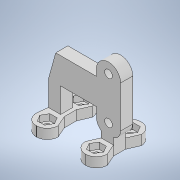
# Autodesk Inventor part: Крепление двигателя
Saved by Autodesk Inventor 2020 (Build 240168000, 168)
## iProperties
Created: 2021-05-24
Part Number: Крепление двигателя
Material: Типовые
Document SubType Name: Modeling
Designer: Антон
Density: 1 g/cm^3
Appearance: По умолчанию
Author: Антон
Autodesk Inventor part; units mm, degrees
ref_plane "YZ Plane" through (0, 0, 0) normal (1, 0, 0) x (0, 1, 0)
ref_plane "XZ Plane" through (0, 0, 0) normal (0, 1, 0) x (-1, 0, 0)
sketch "Эскиз1" plane through (0, 0, 0) normal (0, 0, 1) x (1, 0, 0)
  line L0 (0, 0) -> (26.75, 0)
  line L1 (26.75, 0) -> (26.75, 26)
  line L2 (26.75, 26) -> (0, 26)
  line L3 (0, 26) -> (0, 0)
  line L4 (0, 0) -> (16.75, 0)
  line L5 (16.75, 0) -> (16.75, 7.6)
  line L6 (16.75, 7.6) -> (0, 7.6)
  line L7 (0, 7.6) -> (0, 0)
  line L8 (0, 26) -> (16.75, 26)
  line L9 (16.75, 26) -> (16.75, 18.4)
  line L10 (16.75, 18.4) -> (0, 18.4)
  line L11 (0, 18.4) -> (0, 26)
  point P0 (0, 7.6)
  dimension "d0" = 26.75
  dimension "d1" = 26
  dimension "d14" = 16.75
  dimension "d15" = 7.6
  constraints: 24 end point, 6 parallel, 3 horizontal, 3 perpendicular, 2 equal length
  measures "d0" distance of L2.end L1.end
  measures "d1" distance of L1.end L0.end
  measures "d14" distance of L6.end L5.end
  measures "d15" distance of L5.end L4.end
extrude "Выдавливание1" add sketch "Эскиз1" along normal blind 5 contours L5 L6 L3 L10 L9 L2 L1 L0
sketch "Эскиз2" plane through (0, 0, 5) normal (0, 0, 1) x (1, 0, 0)
  line L0 (26.75, 0) -> (26.75, 26) projected
  line L1 (26.75, 13) -> (21.75, 13)
  line L2 (21.75, 13) -> (21.75, 21.75)
  line L3 (21.75, 13) -> (21.75, 4.25)
  point P0 (0, 0)
  dimension "d4" = 5
  dimension "d6" = 17.5
  constraints: 6 end point, 1 collinear, 1 horizontal, 1 midpoint, 1 perpendicular, 1 vertical
  measures "d4" distance of L1.start L1.end
  measures "d6" distance of L3.end L2.end
hole "Отверстие1" at (21.75, 21.75, 5) at (21.75, 4.25, 5) direction (0, 0, -1) diameter 3.2 end through all
sketch "Эскиз4" plane through (0, 0, 0) normal (0, 0, -1) x (-1, 0, 0)
  line L0 (-23.75, 0) -> (-18.75, 0)
  line L1 (-18.75, 0) -> (-18.75, -6.62)
  line L2 (-18.75, -6.62) -> (-23.75, -6.62)
  line L3 (-23.75, -6.62) -> (-23.75, 0)
  line L4 (3, 7.6) -> (-2, 7.6)
  line L5 (-2, 7.6) -> (-2, -6.62)
  line L6 (-2, -6.62) -> (3, -6.62)
  line L7 (3, -6.62) -> (3, 7.6)
  line L8 (-16.75, 0) -> (-26.75, 0) projected
  line L9 (-26.75, 0) -> (-26.75, 26) projected
  line L10 (0, 7.6) -> (-16.75, 7.6) projected
  line L11 (0, 18.4) -> (0, 7.6) projected
  point P0 (0, 0)
  dimension "d20" = 5
  dimension "d21" = 6.62
  dimension "d22" = 5
  dimension "d82" = 3
  dimension "d83" = 3
  constraints: 16 end point, 4 parallel, 3 collinear, 2 horizontal, 2 perpendicular
  measures "d20" distance of L1.end L2.end
  measures "d21" distance of L0.end L1.end
  measures "d22" distance of L6.end L5.end
  measures "d82" distance between parallel lines of L3 L9
  measures "d83" distance between parallel lines of L11 L7
extrude "Выдавливание3" add sketch "Эскиз4" against normal up to surface (5 mm away)
sketch "Эскиз5" plane through (18.75, -6.62, 0) normal (0, -1, 0) x (1, 0, 0)
  line L0 (7, 0) -> (-2, 0)
  line L1 (-2, 0) -> (-2, -9)
  line L2 (-2, -9) -> (7, -9)
  line L3 (7, -9) -> (7, 0)
  line L4 (5, 0) -> (0, 0) projected
  line L5 (-13.25, 0) -> (-22.25, 0)
  line L6 (-22.25, 0) -> (-22.25, -9)
  line L7 (-22.25, -9) -> (-13.25, -9)
  line L8 (-13.25, -9) -> (-13.25, 0)
  line L9 (-16.75, 0) -> (-18.75, 0) projected
  line L10 (-2, -4.5) -> (7, -4.5)
  line L11 (-13.25, -4.5) -> (-22.25, -4.5)
  circle A0 centre (-17.75, -4.5) radius 1.6
  circle A1 centre (2.5, -4.5) radius 1.6
  point P0 (2.5, 0)
  point P1 (-17.75, 0)
  dimension "d25" = 9
  dimension "d26" = 9
  dimension "d27" = 9
  dimension "d28" = 9
  dimension "d64" = 3.2
  dimension "d65" = 3.2
  constraints: 20 end point, 10 midpoint, 4 parallel, 2 centre point, 2 horizontal, 2 perpendicular
  measures "d25" distance of L2.end L1.end
  measures "d26" distance of L1.end L0.end
  measures "d27" distance of L7.end L6.end
  measures "d28" distance of L6.end L5.end
  measures "d64" diameter of A0
  measures "d65" diameter of A1
extrude "Выдавливание4" add sketch "Эскиз5" against normal blind 4 contours L3 L10 A1 L1 L0 | L3 L2 L1 L10 A1 | L8 L11 A0 L6 L5 | L8 L7 L6 L11 A0
sketch "Эскиз12" plane through (18.75, -2.62, 0) normal (0, 1, 0) x (1, 0, 0)
  circle A0 centre (-17.75, 4.5) radius 1.6 projected
  circle A1 centre (2.5, 4.5) radius 1.6 projected
  line L0 (-16.2489, 7.1) -> (-14.7478, 4.5)
  line L1 (-14.7478, 4.5) -> (-16.2489, 1.9)
  line L2 (-16.2489, 1.9) -> (-19.2511, 1.9)
  line L3 (-19.2511, 1.9) -> (-20.7522, 4.5)
  line L4 (-20.7522, 4.5) -> (-19.2511, 7.1)
  line L5 (-19.2511, 7.1) -> (-16.2489, 7.1)
  line L6 (4.0011, 7.1) -> (5.5022, 4.5)
  line L7 (5.5022, 4.5) -> (4.0011, 1.9)
  line L8 (4.0011, 1.9) -> (0.9989, 1.9)
  line L9 (0.9989, 1.9) -> (-0.5022, 4.5)
  line L10 (-0.5022, 4.5) -> (0.9989, 7.1)
  line L11 (0.9989, 7.1) -> (4.0011, 7.1)
  line L12 (-13.25, 9) -> (-22.25, 9) projected
  line L13 (7, 9) -> (-2, 9) projected
  point P0 (-18.75, 0)
  dimension "d66" = 5.2
  constraints: 24 end point, 2 coincident, 2 parallel, 1 collinear, 26 other
  measures "d66" distance between parallel lines of L5 L2
extrude "Выдавливание10" cut sketch "Эскиз12" against normal blind 2.6 contours A0 | A1 | L0 L1 L2 L3 L4 L5 | L6 L7 L8 L9 L10 L11
fillet "Сопряжение3" radius 4.4685 4 edges at (5.5, -4.62, -9) (-3.5, -4.62, -9) (16.75, -4.62, -9) (25.75, -4.62, -9)
chamfer "Фаска1" distance 4.53 distance2 0.468 1 edges at (-3.5, -4.62, 0) measured on face at (-3.5, -5.2867, -1.5105)
chamfer "Фаска2" distance 1.968 distance2 4.53 1 edges at (25.75, -4.62, 0) measured on face at (25.0833, -5.2867, 0)
chamfer "Фаска3" distance 1.968 distance2 4.53 1 edges at (5.5, -4.62, 0) measured on face at (4.3333, -5.2867, 0)
chamfer "Фаска4" distance 1.968 distance2 4.53 1 edges at (16.75, -4.62, 0) measured on face at (17.4167, -3.9533, 0)
ref_plane "РабПлоскость1" through (0, 0, 2.5) normal (0, 0, -1) x (-1, 0, 0)
mirror "Зеркальное отражение1" about plane through (0, 0, 2.5) normal (0, 0, -1) of "Выдавливание4", "Выдавливание10", "Фаска2", "Фаска4", "Фаска3", "Фаска1", "Сопряжение3"
sketch "Эскиз8" plane through (0, 0, 0) normal (0, 0, -1) x (-1, 0, 0)
  circle A0 centre (-21.75, 21.75) radius 1.6 projected
  line L0 (-23.2511, 19.15) -> (-24.7522, 21.75)
  line L1 (-24.7522, 21.75) -> (-23.2511, 24.35)
  line L2 (-23.2511, 24.35) -> (-20.2489, 24.35)
  line L3 (-20.2489, 24.35) -> (-18.7478, 21.75)
  line L4 (-18.7478, 21.75) -> (-20.2489, 19.15)
  line L5 (-20.2489, 19.15) -> (-23.2511, 19.15)
  circle A1 centre (-21.75, 4.25) radius 1.6 projected
  line L6 (-20.2489, 6.85) -> (-18.7478, 4.25)
  line L7 (-18.7478, 4.25) -> (-20.2489, 1.65)
  line L8 (-20.2489, 1.65) -> (-23.2511, 1.65)
  line L9 (-23.2511, 1.65) -> (-24.7522, 4.25)
  line L10 (-24.7522, 4.25) -> (-23.2511, 6.85)
  line L11 (-23.2511, 6.85) -> (-20.2489, 6.85)
  line L12 (-16.75, 0) -> (-18.75, 0) projected
  line L13 (-26.75, 26) -> (-16.75, 26) projected
  point P0 (0, 0)
  dimension "d42" = 5.2
  constraints: 24 end point, 3 parallel, 2 coincident, 26 other
  measures "d42" distance between parallel lines of L5 L2
hole "Отверстие3" at (21.75, 21.75, 0) at (21.75, 4.25, 0) direction (0, 0, 1) diameter 2.2 end through all counterbore diameter 4 counterbore depth 2
fillet "Сопряжение2" radius 5 3 edges at (26.75, 26, 2.5) (16.75, 26, 2.5) (16.75, 0, 2.5)
fillet "Сопряжение2" radius 4 1 edges at (26.75, 0, 2.5)
chamfer "Фаска5" distance 10.8 distance2 3 1 edges at (0, 7.6, 2.5) measured on face at (0, 14.8, 1.6667)
sketch "Эскиз13" plane through (3.532, -6.62, 5) normal (0, 0, -1) x (-1, 0, 0)
  line L0 (0, 0) -> (0, 4) projected
  line L1 (0, 0) -> (1.532, 0) projected
  line L2 (1.532, 4) -> (1.532, 0) projected
  line L3 (1.532, 4) -> (0, 4) projected
  point P0 (3.532, 6.62)
extrude "Выдавливание11" add sketch "Эскиз13" along normal up to surface (5 mm away)
